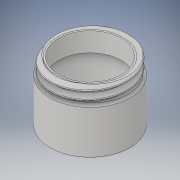
# Autodesk Inventor part: CMF
Saved by Autodesk Inventor 2018 (Build 220112000, 112)
## iProperties
Created: 2017-07-31
Part Number: CMF
Material: Generic
Document SubType Name: Modeling
Designer: Nour Kanso
Density: 1 g/cm^3
Appearance: Default
Mass: 29.9249 g
Surface Area: 270.348 cm^2
Volume: 29.9249 cm^3
Author: Nour Kanso
Autodesk Inventor part; units mm, degrees
ref_plane "YZ Plane" through (0, 0, 0) normal (1, 0, 0) x (0, 1, 0)
ref_plane "XZ Plane" through (0, 0, 0) normal (0, 1, 0) x (-1, 0, 0)
ref_plane "XY Plane" through (0, 0, 0) normal (0, 0, 1) x (1, 0, 0)
sketch "Sketch13" plane through (0, 0, 0) normal (0, 1, 0) x (-1, 0, 0)
  circle A0 centre (0, 0) radius 31.75
  dimension "d72" = 63.5
  constraints: 1 centre point, 1 coincident
  measures "d72" diameter of A0
extrude "Extrusion4" add sketch "Sketch13" along normal blind 2.54
sketch "Sketch14" plane through (0, 2.54, 0) normal (0, 1, 0) x (1, 0, 0)
  circle A0 centre (0, 0) radius 31.75
  constraints: 1 centre point, 1 coincident
extrude "Extrusion5" add sketch "Sketch14" along normal blind 33.02
shell "Shell1" thickness 2.54 removed faces 1 at (1.2757, 35.56, -9.285)
fillet "Fillet2" radius 1.27 1 edges at (31.75, 0, 0)
sketch "Sketch16" plane through (0, 35.56, 0) normal (0, 1, 0) x (1, 0, 0)
  circle A0 centre (0, 0) radius 30.48
  constraints: 1 centre point, 1 coincident
extrude "Extrusion6" add sketch "Sketch16" along normal blind 12.7
sketch "Sketch21" plane through (0, 48.26, 0) normal (0, 1, 0) x (1, 0, 0)
  circle A0 centre (0, 0) radius 29.21
  dimension "d104" = 58.42
  constraints: 1 centre point, 1 coincident
  measures "d104" diameter of A0
extrude "Extrusion8" cut sketch "Sketch21" against normal blind 45.72
thread "Thread6" size "2 1/2-4 UNC" class "2A" standard "ANSI Unified Screw Threads" full length
sketch "Sketch26" plane through (0, 48.26, 0) normal (1, 0, 0) x (0, 0, 1)
  line L0 (30.48, 0) -> (30.48, 12.7)
  line L1 (30.48, 12.7) -> (26.3361, 12.7)
  line L2 (26.3361, 12.7) -> (26.3361, 0)
  line L3 (26.3361, 0) -> (30.48, 0)
  line L4 (0, -42.5335) -> (0, 63.3922) projected
  constraints: 8 end point
revolve "Revolution11" cut sketch "Sketch26" angle 360 about axis through (0, 48.26, 0) along (0, -1, 0)
sketch "Sketch27" plane through (0, 48.26, 0) normal (1, 0, 0) x (0, 0, 1)
  line L0 (30.48, 0) -> (30.48, 12.7)
  line L1 (30.48, 12.7) -> (26.3361, 12.7)
  line L2 (26.3361, 12.7) -> (26.3361, 0)
  line L3 (26.3361, 0) -> (30.48, 0)
  line L4 (0, -42.5335) -> (0, 63.3922) projected
  constraints: 8 end point
revolve "Revolution12" add sketch "Sketch27" angle 360 about axis through (0, 48.26, 0) along (0, -1, 0) separate body
sketch "Sketch25" plane through (0, 48.26, 0) normal (-1, 0, 0) x (0, -1, 0)
  line L0 (-3.762, -26.6751) -> (-3.1751, -26.6751) construction
  line L1 (0.5868, -30.1413) -> (-0.0001, -31.1579) construction
  line L2 (-6.3501, -31.1579) -> (-6.937, -30.1413) construction
  line L3 (-2.5882, -26.6751) -> (-3.1751, -25.6586) construction
  line L4 (-3.1751, -25.6586) -> (-3.762, -26.6751) construction
  line L5 (-6.3501, -31.1579) -> (-5.7632, -30.1413) construction
  line L6 (-2.5882, -26.6751) -> (-0.587, -30.1413)
  line L7 (-6.937, -30.1413) -> (-5.7632, -30.1413) construction
  arc A0 (-6.937, -30.1413) -> (-6.3501, -30.4802) centre (-6.3501, -29.8025) ccw construction
  line L8 (0.5868, -30.1413) -> (-0.587, -30.1413) construction
  line L9 (-6.3501, -31.1579) -> (-6.3501, -30.1413) construction
  line L10 (-0.0001, -31.1579) -> (-0.0001, -30.1413) construction
  line L11 (-3.1751, -25.6586) -> (-3.1751, -26.3363) construction
  line L12 (-6.3501, -30.4802) -> (-0.0001, -30.4802)
  arc A1 (-6.3501, -30.4802) -> (-5.7632, -30.1413) centre (-6.3501, -29.8025) ccw
  line L13 (-0.587, -30.1413) -> (-0.0001, -31.1579) construction
  line L14 (-5.7632, -30.1413) -> (-3.762, -26.6751)
  line L15 (-0.0001, -0.0002) -> (-0.0001, 0.0177)
  line L16 (-0.0001, 0.0177) -> (-0.0001, -0.0002)
  line L17 (-0.0001, -0.0002) -> (0.0334, -0.0002)
  arc A2 (-0.587, -30.1413) -> (-0.0001, -30.4802) centre (-0.0001, -29.8025) ccw
  arc A3 (-0.0001, -30.4802) -> (0.5868, -30.1413) centre (-0.0001, -29.8025) ccw construction
  arc A4 (-3.1751, -26.3363) -> (-3.762, -26.6751) centre (-3.1751, -27.014) ccw
  arc A5 (-2.5882, -26.6751) -> (-3.1751, -26.3363) centre (-3.1751, -27.014) ccw
  line L18 (-3.1751, -26.3363) -> (-3.1751, -26.6751) construction
  line L19 (-3.1751, -26.6751) -> (-2.5882, -26.6751) construction
  dimension "d130" = 60
  dimension "d131" = 1.0165
  dimension "d132" = 1.0165
  dimension "Sketch25_ThreadOffset" = 0
  dimension "Sketch25_MajorRadius" = 30.48
  dimension "d135" = 6.35
  dimension "Sketch25_MinorRadius" = 26.3361
  constraints: 40 end point, 12 point on circle, 10 parallel, 8 tangent, 6 centre point, 6 collinear, 2 midpoint, 2 point on line, 1 horizontal, 1 perpendicular, 3 other
  measures "d130" angle of L6 L14
  measures "d131" distance of L3.end L0.end
  measures "d132" distance of L1.end L10.end
  measures "Sketch25_ThreadOffset" distance between parallel lines of L15 L10
  measures "Sketch25_MajorRadius" distance from line of L12 L15.start
  measures "d135" distance from line of L1.end L9
  measures "Sketch25_MinorRadius" distance edge to line of A5 L17
coil "Coil6" sketch "Sketch25" operation cut axis through (0, 48.26, 0) along (0, -1, 0) pitch 6.3563 turns 3.996004 hand right bodies 2
sketch "Sketch33" plane through (0, 35.56, 0) normal (0, 1, 0) x (1, 0, 0)
  circle A0 centre (0, 0) radius 30.48
  dimension "d161" = 60.96
  constraints: 1 centre point, 1 coincident
  measures "d161" diameter of A0
extrude "Extrusion14" cut sketch "Sketch33" against normal blind 33.02 bodies 1
sketch "Sketch34" plane through (0, 35.56, 0) normal (0, 1, 0) x (1, 0, 0)
  circle A0 centre (0, 0) radius 30.48
  constraints: 1 centre point, 1 coincident
extrude "Extrusion15" add sketch "Sketch34" against normal blind 2.54 bodies 1
sketch "Sketch35" plane through (0, 35.56, 0) normal (0, 1, 0) x (1, 0, 0)
  circle A0 centre (0, 0) radius 25.0698
  dimension "d166" = 50.1396
  constraints: 1 centre point, 1 coincident
  measures "d166" diameter of A0
extrude "Extrusion16" cut sketch "Sketch35" against normal blind 2.54 bodies 1
sketch "Sketch36" plane through (0, 35.56, 0) normal (0, 1, 0) x (1, 0, 0)
  circle A0 centre (0, 0) radius 26.3361
  constraints: 1 centre point, 1 coincident
extrude "Extrusion17" add sketch "Sketch36" along normal blind 12.7 bodies 1
sketch "Sketch37" plane through (0, 48.26, 0) normal (0, 1, 0) x (1, 0, 0)
  circle A0 centre (0, 0) radius 25.0698
  dimension "d171" = 50.1396
  constraints: 1 centre point, 1 coincident
  measures "d171" diameter of A0
extrude "Extrusion18" cut sketch "Sketch37" against normal blind 12.7 bodies 1
equation "\"d130\" = d137"
equation "\"d131\" = 0.160083 * Sketch25_Pitch"
equation "\"d132\" = 0.160083 * Sketch25_Pitch"
equation "\"d135\" = Sketch25_Pitch"
equation "\"d17\" = 60deg"
equation "\"Sketch4_Pitch\" = 6.35"
equation "\"d39\" = 60deg"
equation "\"Sketch7_Pitch\" = 6.35"
equation "\"d60\" = 60deg"
equation "\"Sketch10_Pitch\" = 6.35"
equation "\"d92\" = 60deg"
equation "\"Sketch18_Pitch\" = 6.35"
equation "\"d116\" = 60deg"
equation "\"Sketch22_Pitch\" = 6.35"
equation "\"d137\" = 60deg"
equation "\"Sketch25_Pitch\" = 6.35"
body "Solid5"
body "Solid8"
